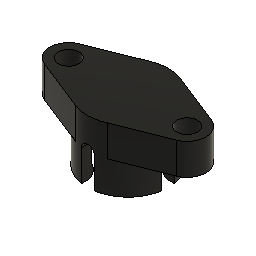
Caster Holder (Autodesk Fusion 360 design; units mm, degrees)
Autodesk Fusion 360 part; units mm, degrees
note: some values were not read from the file. Set by a fixed rule: which sketch regions a step uses.
sketch "Sketch1" plane through (0, 0, 0) normal (0, 1, 0) x (1, 0, 0)
  arc A0 (-4.719, 7.6667) -> (-1.5623, 1.2487) centre (-0.005, 6) ccw
  line L0 (-6.505, -1) -> (-6.505, 9)
  line L1 (0, -1) -> (-6.505, -1)
  line L2 (0, -1) -> (0, 2)
  line L3 (-0.9983, 4) -> (-0.9983, 9.5)
  line L4 (1.0017, 4) -> (1.0017, 9.5)
  line L5 (-0.9983, 9.5) -> (1.0017, 9.5)
  arc A1 (-0.9983, 4) -> (1.0017, 4) centre (0.0017, 4) ccw
  arc A2 (0, 2) -> (-1.5623, 1.2487) centre (0, 0) ccw
  line L6 (-5.6618, 9) -> (-6.505, 9)
  arc A3 (-4.719, 7.6667) -> (-5.6618, 9) centre (-5.6618, 8) ccw
  dimension "d22" = 5
  dimension "d25" = 4
  dimension "d26" = 2
  dimension "d28" = 1
  dimension "d29" = 7
  dimension "d30" = 1
  dimension "d31" = 0.5
  measures "d22" radius of A0
  measures "d28" radius of A3
  measures "d30" radius of A1
  measures "d31" distance of L5 L6
revolve "Revolve1" add sketch "Sketch1" angle 360 about axis through (0, 0, 1.75) along (0, 0, 1) contours A0 L0 L1 L2 A2 L6 A3
sketch "Sketch4" plane through (0, 0, 1) normal (0, 0, 1) x (-1, 0, 0)
  circle A0 centre (0, 0) radius 6.505
  line L0 (10.604, -2.7795) -> (2.4064, -6.0435)
  line L1 (10.5995, 2.7966) -> (2.3966, 6.0474)
  arc A1 (6.5014, 0.2158) -> (6.5018, -0.2053) centre (9.4942, 0.0077) ccw
  arc A2 (10.604, -2.7795) -> (10.5995, 2.7966) centre (9.4942, 0.0077) ccw
  circle A3 centre (9.4942, 0.0077) radius 1.65
  line L2 (0.0068, -8) -> (0.0068, 8)
  line L3 (-10.5859, 2.7966) -> (-2.383, 6.0474)
  arc A4 (-10.5859, 2.7966) -> (-10.5904, -2.7795) centre (-9.4806, 0.0077) ccw
  circle A5 centre (-9.4806, 0.0077) radius 1.65
  line L4 (-10.5904, -2.7795) -> (-2.3928, -6.0435)
  dimension "d10" = 6
  dimension "d11" = 3.3
  measures "d10" diameter of A1
  measures "d11" diameter of A3
extrude "Extrude1" add sketch "Sketch4" against normal blind 5 contours A0 L0 L1 A2 | A0 L3 A4 L4
extrude "Extrude2" cut sketch "Sketch1" along normal blind 7 contours L3 L4 L5 A1
pattern_circular "C-Pattern1" count 4 over 360 about axis through (0, 0, 1.75) along (0, 0, 1) of "Extrude2"
equation "d25 = d22 - 1 mm"
equation "d26 = d25 / 2"
named bodies: "Caster Housing"
